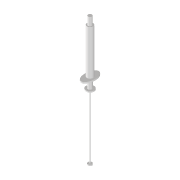
# Autodesk Inventor part: 00_Syringe_10ml
Saved by Autodesk Inventor 2022 (Build 260153000, 153)
## iProperties
Created: 2022-01-10
Part Number: 00_Syringe_10ml
Material: Generisch
Document SubType Name: Modeling
Designer: diederichbenedict
Density: 1 g/cm^3
Appearance: Vorgabe
Author: diederichbenedict
Autodesk Inventor part; units mm, degrees
ref_plane "YZ Plane" through (0, 0, 0) normal (1, 0, 0) x (0, 1, 0)
ref_plane "XZ Plane" through (0, 0, 0) normal (0, 1, 0) x (-1, 0, 0)
ref_plane "XY Plane" through (0, 0, 0) normal (0, 0, 1) x (1, 0, 0)
sketch "Skizze1" plane through (0, 0, 0) normal (0, 1, 0) x (-1, 0, 0)
  circle A0 centre (0, 0) radius 3.22
  dimension "d0" = 6.44
  constraints: 1 centre point, 1 coincident
  measures "d0" diameter of A0
extrude "Extrusion1" add sketch "Skizze1" along normal blind 47.6
sketch "Skizze2" plane through (0, 47.6, 0) normal (0, 1, 0) x (1, 0, 0)
  circle A0 centre (0, 0) radius 3.22 projected
  circle A1 centre (0, 0) radius 3.22 projected
  circle A2 centre (0, 0) radius 2.05
  dimension "d3" = 4.1
  constraints: 1 centre point, 1 coincident
  measures "d3" diameter of A2
extrude "Extrusion2" add sketch "Skizze2" along normal blind 8.5 contours A2
sketch "Skizze3" plane through (0, 0, 0) normal (0, -1, 0) x (1, 0, 0)
  circle A0 centre (0, 0) radius 3.22 projected
  ellipse E0 centre (0, 0) end of major axis (0, -9.5) minor radius 5.25
  line L0 (0, 9.5) -> (0, 0)
  line L1 (0, -10.6353) -> (0, 10.6353) projected
  line L2 (0, 0) -> (-5.25, 0)
  dimension "d6" = 9.5
  dimension "d7" = 5.25
  constraints: 4 end point, 2 coincident, 1 collinear, 1 horizontal, 4 other
  measures "d6" distance of point (0, 0) L0.start
  measures "d7" distance of L2.end point (0, 0)
extrude "Extrusion3" add sketch "Skizze3" along normal blind 1.5
sketch "Skizze4" plane through (0, -1.5, 0) normal (0, -1, 0) x (1, 0, 0)
  circle A0 centre (0, 0) radius 3.22 projected
  circle A1 centre (0, 0) radius 2.165
  dimension "d10" = 4.33
  constraints: 1 centre point, 1 coincident
  measures "d10" diameter of A1
extrude "Extrusion4" add sketch "Skizze4" along normal blind 9.5 contours A1
sketch "Skizze5" plane through (0, -11, 0) normal (0, -1, 0) x (1, 0, 0)
  circle A0 centre (0, 0) radius 2.165 projected
  circle A1 centre (0, 0) radius 4.3
  dimension "d13" = 8.6
  constraints: 1 centre point, 1 coincident
  measures "d13" diameter of A1
extrude "Extrusion5" add sketch "Skizze5" along normal blind 1.2 contours A0 | A1
sketch "Skizze6" plane through (0, -12.2, 0) normal (0, -1, 0) x (1, 0, 0)
  ellipse E0 centre (0, 0) end of major axis (0, -9.5) minor radius 5.25 projected
  circle A0 centre (0, 0) radius 0.5
  dimension "d16" = 1
  constraints: 1 centre point, 1 coincident, 1 other
  measures "d16" diameter of A0
extrude "Extrusion6" add sketch "Skizze6" along normal blind 68.2 contours A0
sketch "Skizze7" plane through (0, -80.4, 0) normal (0, -1, 0) x (1, 0, 0)
  circle A0 centre (0, 0) radius 2.165 projected
extrude "Extrusion7" add sketch "Skizze7" along normal blind 1.2
